# Autodesk Inventor part: 6SLX45TFGG484
Saved by Autodesk Inventor 2015 SP1 (Build 190203100, 203)
## iProperties
Created: 2015-06-25
Part Number: 6SLX45TFGG484
Material: Generic
Document SubType Name: Modeling
Designer: Patrick
Density: 1 g/cm^3
Appearance: FG484, 6SLX45TFGG484
Author: Patrick
Autodesk Inventor part; units mm, degrees
ref_plane "YZ Plane" through (0, 0, 0) normal (1, 0, 0) x (0, 1, 0)
ref_plane "XZ Plane" through (0, 0, 0) normal (0, 1, 0) x (-1, 0, 0)
ref_plane "XY Plane" through (0, 0, 0) normal (0, 0, 1) x (1, 0, 0)
sketch "FG484, 6SLX45TFGG484_8" plane through (0, 0, 0) normal (0, 0, 1) x (1, 0, 0)
  line L0 (-11.5, -11.5) -> (-11.5, 11.5)
  line L1 (-11.5, 11.5) -> (11.5, 11.5)
  line L2 (11.5, 11.5) -> (11.5, -11.5)
  line L3 (11.5, -11.5) -> (-11.5, -11.5)
  constraints: 8 end point
extrude "Extrusion1" add sketch "FG484, 6SLX45TFGG484_8" along normal blind 1
body "Solid1"
